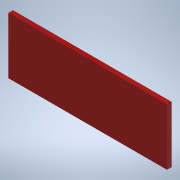
# Autodesk Inventor part: SP46V1 Felpa Roldana
Saved by Autodesk Inventor 2021.2 (Build 252289000, 289)
## iProperties
Created: 2026-09-01
Part Number: SP46V1 Felpa Roldana
Material: Fabric
Document SubType Name: Modeling
Designer: nelso
Density: 0.9 g/cm^3
Appearance: Smooth - Red
Author: nelso
Autodesk Inventor part; units mm, degrees
ref_plane "YZ Plane" through (0, 0, 0) normal (1, 0, 0) x (0, 1, 0)
ref_plane "XZ Plane" through (0, 0, 0) normal (0, 1, 0) x (-1, 0, 0)
ref_plane "XY Plane" through (0, 0, 0) normal (0, 0, 1) x (1, 0, 0)
sketch "Sketch1" plane through (0, 0, 0) normal (0, 1, 0) x (-1, 0, 0)
  line L0 (35, 12.5) -> (-35, 12.5)
  line L1 (-35, 12.5) -> (-35, -12.5)
  line L2 (-35, -12.5) -> (35, -12.5)
  line L3 (35, -12.5) -> (35, 12.5)
  line L4 (35, 12.5) -> (-35, -12.5) construction
  line L5 (-35, 12.5) -> (35, -12.5) construction
  point P0 (0, 0)
  dimension "d0" = 70
  dimension "d1" = 25
  constraints: 12 end point, 2 midpoint, 2 parallel, 1 horizontal, 1 perpendicular
  measures "d0" distance of L2.end L1.end
  measures "d1" distance of L1.end L0.end
extrude "Extrusion1" add sketch "Sketch1" along normal blind 2
body "Solid1"
